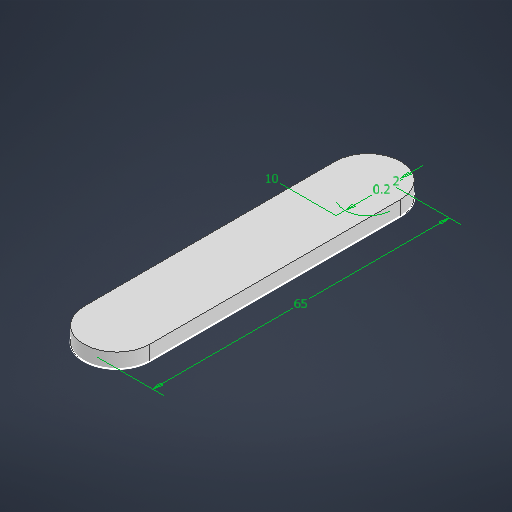
# Autodesk Inventor part: magnet_holder
Saved by Autodesk Inventor 2026.2 (Build 302298000, 298)
## iProperties
Created: 2026-03-09
Part Number: magnet_holder
Material: Generic
Document SubType Name: Modeling
Designer: Tathagata Sikdar
Density: 1 g/cm^3
Appearance: Default
Author: Tathagata Sikdar
Autodesk Inventor part; units mm, degrees
ref_plane "YZ Plane" through (0, 0, 0) normal (1, 0, 0) x (0, 1, 0)
ref_plane "XZ Plane" through (0, 0, 0) normal (0, 1, 0) x (-1, 0, 0)
ref_plane "XY Plane" through (0, 0, 0) normal (0, 0, 1) x (1, 0, 0)
sketch "Sketch1" plane through (0, 0, 0) normal (0, 1, 0) x (-1, 0, 0)
  line L0 (0, 0) -> (0, -65) construction
  line L1 (-5, -5) -> (-5, -60) construction
  line L2 (5, -60) -> (5, -5) construction
  arc A0 (5, -5) -> (-5, -5) centre (0, -5) ccw construction
  arc A1 (-5, -60) -> (5, -60) centre (0, -60) ccw construction
  line L3 (5.2, -60) -> (5.2, -5)
  arc A2 (5.2, -5) -> (-5.2, -5) centre (0, -5) ccw
  line L4 (-5.2, -5) -> (-5.2, -60)
  arc A3 (-5.2, -60) -> (5.2, -60) centre (0, -60) ccw
  line L5 (7.2, -60) -> (7.2, -5)
  arc A4 (7.2, -5) -> (-7.2, -5) centre (0, -5) ccw
  line L6 (-7.2, -5) -> (-7.2, -60)
  arc A5 (-7.2, -60) -> (7.2, -60) centre (0, -60) ccw
  point P0 (0, -32.5)
  dimension "d0" = 65
  dimension "d1" = 10
  dimension "d2" = 0.2
  dimension "d3" = 2
  constraints: 16 end point, 14 point on circle, 6 centre point, 4 tangent, 3 parallel, 2 point on line, 1 midpoint, 1 vertical, 6 other
  measures "d0" distance of L0.start L0.end
  measures "d1" diameter of A1
  measures "d2" radial gap between concentric circles of A1 A3
  measures "d3" radial gap between concentric circles of A3 A5
extrude "Extrusion1" add sketch "Sketch1" along normal blind 2.2
extrude "Extrusion2" add sketch "Sketch1" along normal blind 1 from surface at 2.2 contours A3 L4 A2 L3 | A5 L6 A4 L5
body "Solid1"
